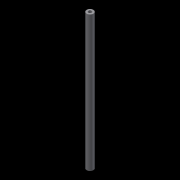
# Autodesk Inventor part: 3d_LM - Tubo 1x1-3
Saved by Autodesk Inventor 2018 (Build 220112000, 112)
## iProperties
Created: 2025-09-03
Part Number: 3d_LM - Tubo 1x1-3
Material: Genérico
Document SubType Name: Modeling
Designer: mbs18
Density: 1 g/cm^3
Appearance: Valor por defecto
Mass: 0.0975665 g
Surface Area: 3.96237 cm^2
Volume: 0.0975665 cm^3
Author: mbs18
Autodesk Inventor part; units mm, degrees
ref_plane "YZ Plane" through (0, 0, 0) normal (1, 0, 0) x (0, 1, 0)
ref_plane "XZ Plane" through (0, 0, 0) normal (0, 1, 0) x (-1, 0, 0)
ref_plane "XY Plane" through (0, 0, 0) normal (0, 0, 1) x (1, 0, 0)
sketch "Sketch1" plane through (0, 0, 0) normal (0, 0, 1) x (1, 0, 0)
  circle A0 centre (0, 0) radius 1
  circle A1 centre (0, 0) radius 0.5
  dimension "d0" = 2
  dimension "d1" = 1
  constraints: 2 centre point, 2 coincident
  measures "d0" diameter of A0
  measures "d1" diameter of A1
extrude "Extrusion1" add sketch "Sketch1" along normal blind 40
body "Solid1"
